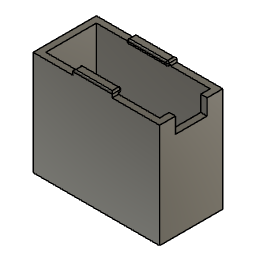
samsung-psu-holder (Autodesk Fusion 360 design; units mm, degrees)
Autodesk Fusion 360 part; units mm, degrees
sketch "Skizze1" plane through (0, 0, 0) normal (0, 0, 1) x (1, 0, 0)
  line L0 (0, 0) -> (80, 0)
  line L1 (80, 0) -> (80, -40)
  line L2 (80, -40) -> (0, -40)
  line L3 (0, -40) -> (0, 0)
  line L4 (76, -36) -> (4, -36)
  line L5 (4, -36) -> (4, -4)
  line L6 (4, -4) -> (76, -4)
  line L7 (76, -4) -> (76, -36)
  dimension "d1" = 80
  dimension "d2" = 40
  dimension "d3" = 4
  constraint horizontal L0
  constraint vertical L1
  constraint horizontal L2
  constraint vertical L3
  constraint coincident L0.start L3.end
  measures "d1" distance of L0.start L0.end
  measures "d2" distance of L0.start L2.end
extrude "Extrusion1" add sketch "Skizze1" along normal blind 4 contours L4 L5 L6 L7
sketch "Skizze2" plane through (0, 0, 0) normal (0, 0, 1) x (1, 0, 0)
  line L0 (0, 0) -> (80, 0)
  line L1 (80, 0) -> (80, -40)
  line L2 (80, -40) -> (0, -40)
  line L3 (0, -40) -> (0, 0)
  line L4 (76, -4) -> (76, -36)
  line L5 (76, -36) -> (4, -36)
  line L6 (4, -36) -> (4, -4)
  line L7 (4, -4) -> (76, -4)
  dimension "d6" = 80
  dimension "d7" = 40
  dimension "d8" = 4
  constraint horizontal L0
  constraint vertical L1
  constraint horizontal L2
  constraint vertical L3
  constraint coincident L0.start L3.end
  measures "d6" distance of L0.start L0.end
  measures "d7" distance of L0.start L2.end
extrude "Extrusion2" add sketch "Skizze2" along normal blind 66
sketch "Skizze3" plane through (0, 0, 66) normal (0, 0, 1) x (-1, 0, 0)
  line L0 (-4, 36) -> (-4, 4)
  line L1 (-4, 4) -> (-76, 4)
  line L2 (-76, 4) -> (-76, 36)
  line L3 (-76, 36) -> (-4, 36)
  line L4 (0, 40) -> (-80, 40)
  line L5 (-80, 40) -> (-80, 0)
  line L6 (-80, 0) -> (0, 0)
  line L7 (0, 0) -> (0, 40)
  line L8 (-76, 9.9367) -> (-80, 9.9367)
  line L9 (-80, 9.9367) -> (-80, 29.9367)
  line L10 (-80, 29.9367) -> (-76, 29.9367)
  line L11 (-76, 29.9367) -> (-76, 9.9367)
  dimension "d11" = 4
  dimension "d12" = 20
  constraint horizontal L8
  constraint vertical L9
  constraint horizontal L10
  constraint vertical L11
  constraint coincident L2 L8.start
  measures "d11" distance of L8.start L8.end
  measures "d12" distance of L8.start L10.end
extrude "Extrusion3" cut sketch "Skizze3" against normal blind 10 contours L2 L5 L8 L9 L10 L11
sketch "Skizze4" plane through (0, 0, 66) normal (0, 0, 1) x (-1, 0, 0)
  line L0 (-80, 29.9367) -> (-76, 29.9367)
  line L1 (-76, 29.9367) -> (-76, 36)
  line L2 (-76, 36) -> (-4, 36)
  line L3 (-4, 36) -> (-4, 4)
  line L4 (-4, 4) -> (-76, 4)
  line L5 (-76, 4) -> (-76, 9.9367)
  line L6 (-76, 9.9367) -> (-80, 9.9367)
  line L7 (-80, 9.9367) -> (-80, 0)
  line L8 (-80, 0) -> (0, 0)
  line L9 (0, 0) -> (0, 40)
  line L10 (0, 40) -> (-80, 40)
  line L11 (-80, 40) -> (-80, 29.9367)
  line L12 (-25, 0) -> (-51, 0)
  line L13 (-51, 0) -> (-51, 6)
  line L14 (-51, 6) -> (-25, 6)
  line L15 (-25, 6) -> (-25, 0)
  dimension "d15" = 26
  constraint horizontal L12
  constraint vertical L13
  constraint horizontal L14
  constraint vertical L15
  constraint coincident L8 L12.start
  measures "d15" distance of L12.start L12.end
extrude "Extrusion4" add sketch "Skizze4" along normal blind 3 contours L4 L8 L12 L13 L15 | L4 L13 L14 L15
sketch "Skizze5" plane through (0, 0, 66) normal (0, 0, 1) x (-1, 0, 0)
  line L0 (-25, 4) -> (-25, 0)
  line L1 (-25, 0) -> (0, 0)
  line L2 (0, 0) -> (0, 40)
  line L3 (0, 40) -> (-80, 40)
  line L4 (-80, 40) -> (-80, 29.9367)
  line L5 (-80, 29.9367) -> (-76, 29.9367)
  line L6 (-76, 29.9367) -> (-76, 36)
  line L7 (-76, 36) -> (-4, 36)
  line L8 (-4, 36) -> (-4, 4)
  line L9 (-4, 4) -> (-25, 4)
  line L10 (-25, 40) -> (-50, 40)
  line L11 (-50, 40) -> (-50, 34)
  line L12 (-50, 34) -> (-25, 34)
  line L13 (-25, 34) -> (-25, 40)
  dimension "d18" = 25
  dimension "d19" = 6
  constraint horizontal L10
  constraint vertical L11
  constraint horizontal L12
  constraint vertical L13
  constraint coincident L3 L10.start
  measures "d18" distance of L10.start L10.end
  measures "d19" distance of L10.start L12.end
extrude "Extrusion5" add sketch "Skizze5" along normal blind 3 contours L7 L11 L12 L13 | L3 L7 L10 L11 L13
fillet "Abrundung1" radius 1 18 edges at (38, -6, 69) (51, -6, 67.5) (25, -6, 67.5) (38, -6, 66) (51, -3, 69) (37.5, -40, 69) (50, -37, 69) (50, -34, 67.5) (37.5, -34, 69) (25, -37, 69) (25, -3, 69) (25, -34, 67.5) (37.5, -34, 66) (25, -35, 66) (51, -5, 66) (50, -35, 66) (25, -5, 66) (38, 0, 69)
